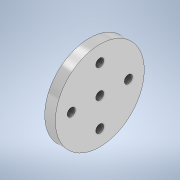
# Autodesk Inventor part: Part L
Saved by Autodesk Inventor 2021 (Build 250183000, 183)
## iProperties
Created: 2021-10-22
Part Number: Part L
Material: Generic
Document SubType Name: Modeling
Designer: Asus
Density: 1 g/cm^3
Appearance: Default
Author: Asus
Autodesk Inventor part; units mm, degrees
ref_plane "YZ Plane" through (0, 0, 0) normal (1, 0, 0) x (0, 1, 0)
ref_plane "XZ Plane" through (0, 0, 0) normal (0, 1, 0) x (-1, 0, 0)
ref_plane "XY Plane" through (0, 0, 0) normal (0, 0, 1) x (1, 0, 0)
sketch "Sketch1" plane through (0, 0, 0) normal (1, 0, 0) x (0, 1, 0)
  circle A0 centre (0, 0) radius 10.9
  dimension "d0" = 21.8
  constraints: 1 centre point, 1 coincident
  measures "d0" diameter of A0
extrude "Extrusion1" add sketch "Sketch1" along normal blind 2.6
sketch "Sketch2" plane through (0, 0, 0) normal (-1, 0, 0) x (0, 0, 1)
  circle A0 centre (0, 0) radius 2.5
  circle A1 centre (0, 0) radius 3.5
  dimension "d3" = 5
  dimension "d4" = 7
  constraints: 2 centre point, 2 coincident
  measures "d3" diameter of A0
  measures "d4" diameter of A1
extrude "Extrusion2" add sketch "Sketch2" along normal blind 2.2
sketch "Sketch3" plane through (2.6, 0, 0) normal (1, 0, 0) x (0, 0, -1)
  circle A0 centre (0, 0) radius 1
  dimension "d7" = 2
  constraints: 1 centre point, 1 coincident
  measures "d7" diameter of A0
hole "Hole1" at (2.6, 0, 0) direction (-1, 0, 0) diameter 2 depth 2
thread "Thread1" size "M2x0.4" class "6H" standard "ANSI Metric M Profile" length 5
sketch "Sketch4" plane through (2.6, 0, 0) normal (1, 0, 0) x (0, 0, -1)
  circle A0 centre (0, 0) radius 1 projected
  circle A1 centre (0, 0) radius 7
  circle A2 centre (-7, 0) radius 1
  circle A3 centre (0, -7) radius 1
  circle A4 centre (7, 0) radius 1
  circle A5 centre (0, 7) radius 1
  dimension "d17" = 14
  dimension "d18" = 2
  dimension "d21" = 360
  constraints: 4 centre point, 1 coincident, 1 horizontal alignment, 11 other
  measures "d18" diameter of A2
hole "Hole2" at (2.6, -7, 0) at (2.6, 0, 7) at (2.6, 7, 0) at (2.6, 0, -7) at (2.6, 0, 0) direction (-1, 0, 0) diameter 2 depth 3
thread "Thread2" size "M2x0.4" class "6H" standard "ANSI Metric M Profile" length 4
thread "Thread3" size "M2x0.4" class "6H" standard "ANSI Metric M Profile" length 4
thread "Thread4" size "M2x0.4" class "6H" standard "ANSI Metric M Profile" length 4
thread "Thread5" size "M2x0.4" class "6H" standard "ANSI Metric M Profile" length 4
body "Solid1"
